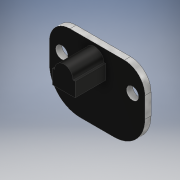
# Autodesk Inventor part: TSSP Board
Saved by Autodesk Inventor 2018 (Build 220112000, 112)
## iProperties
Created: 2018-09-04
Part Number: TSSP Board
Material: Generic
Document SubType Name: Modeling
Designer: matth
Density: 1 g/cm^3
Appearance: Default
Author: matth
Autodesk Inventor part; units mm, degrees
ref_plane "YZ Plane" through (0, 0, 0) normal (1, 0, 0) x (0, 1, 0)
ref_plane "XZ Plane" through (0, 0, 0) normal (0, 1, 0) x (-1, 0, 0)
ref_plane "XY Plane" through (0, 0, 0) normal (0, 0, 1) x (1, 0, 0)
sketch "Sketch1" plane through (0, 0, 0) normal (0, 1, 0) x (-1, 0, 0)
  line L0 (0, 0) -> (8, 0)
  line L1 (0, 0) -> (-9.27, 0)
  circle A0 centre (8, 0) radius 1.5
  circle A1 centre (-9.27, 0) radius 1.5
  line L2 (8, 0) -> (11, 0)
  line L3 (-9.27, 0) -> (-12.27, 0)
  line L4 (11, 0) -> (11, 6)
  line L5 (-12.27, 0) -> (-12.27, -11.5)
  line L6 (11, 6) -> (-12.27, 6)
  line L7 (-12.27, 6) -> (-12.27, -11.5)
  line L8 (-12.27, -11.5) -> (11, -11.5)
  line L9 (11, -11.5) -> (11, 6)
  dimension "d0" = 8
  dimension "d1" = 9.27
  dimension "d2" = 3
  dimension "d3" = 3
  dimension "d4" = 3
  dimension "d5" = 3
  dimension "d6" = 6
  dimension "d7" = 11.5
  constraints: 20 end point, 5 horizontal, 2 centre point, 2 coincident, 2 parallel, 2 vertical, 1 perpendicular
  measures "d0" distance of L0.start L0.end
  measures "d1" distance of L0.start L1.end
  measures "d2" diameter of A0
  measures "d3" diameter of A1
  measures "d4" distance of L2.start L2.end
  measures "d5" distance of L3.start L3.end
  measures "d6" distance of L2.end L4.end
  measures "d7" distance of L3.end L5.end
extrude "Extrusion1" add sketch "Sketch1" along normal blind 1.5 contours L1 A1 L3 L7 L6 L4 L2 A0 L0 | L0 A0 L2 L9 L8 L5 L3 A1 L1
fillet "Fillet1" radius 5 2 edges at (-11, 0.75, 6) (12.27, 0.75, 6)
fillet "Fillet2" radius 7.5 2 edges at (-11, 0.75, -11.5) (12.27, 0.75, -11.5)
sketch "Sketch2" plane through (0, 1.5, 0) normal (0, 1, 0) x (1, 0, 0)
  line L0 (4.77, 11.5) -> (-3.5, 11.5) projected
  line L1 (0, 11.5) -> (2, 11.5)
  line L2 (2, 11.5) -> (0, 11.5)
  line L3 (0, 11.5) -> (0, 9.5)
  line L4 (0, 9.5) -> (-5, 9.5)
  line L5 (-5, 9.5) -> (5, 9.5)
  line L6 (5, 9.5) -> (5, 4.5)
  line L7 (5, 4.5) -> (-5, 4.5)
  line L8 (-5, 4.5) -> (-5, 9.5)
  point P0 (0, 0)
  dimension "d12" = 2
  dimension "d13" = 2
  dimension "d14" = 5
  dimension "d15" = 10
  dimension "d16" = 5
  constraints: 16 end point, 3 equal length, 3 perpendicular, 2 point on line, 1 horizontal
  measures "d12" distance of L1.start L1.end
  measures "d13" distance of L1.start L3.end
  measures "d14" distance of L3.end L4.end
  measures "d15" distance of L6.end L7.end
  measures "d16" distance of L5.end L6.end
extrude "Extrusion2" add sketch "Sketch2" along normal blind 2.5
sketch "Sketch3" plane through (0, 0, 0) normal (0, -1, 0) x (1, 0, 0)
  line L0 (0, 0) -> (0, -0.48)
  line L1 (0, -0.48) -> (2.75, -0.48)
  line L2 (2.75, -0.48) -> (2.75, 3.02)
  line L3 (2.75, 3.02) -> (-2.75, 3.02)
  line L4 (-2.75, 3.02) -> (-2.75, -0.48)
  line L5 (-2.75, -0.48) -> (0, -0.48)
  circle A0 centre (0, 3.02) radius 2.25
  dimension "d19" = 0.48
  dimension "d20" = 2.75
  dimension "d21" = 3.5
  dimension "d22" = 5.5
  dimension "d23" = 4.5
  constraints: 12 end point, 3 perpendicular, 1 centre point, 1 collinear, 1 horizontal, 1 midpoint, 1 point on line, 1 vertical
  measures "d19" distance of L0.start L0.end
  measures "d20" distance of L0.end L1.end
  measures "d21" distance of L1.end L2.end
  measures "d22" distance of L2.end L3.end
  measures "d23" diameter of A0
extrude "Extrusion3" add sketch "Sketch3" along normal blind 7.5
body "Solid1"
